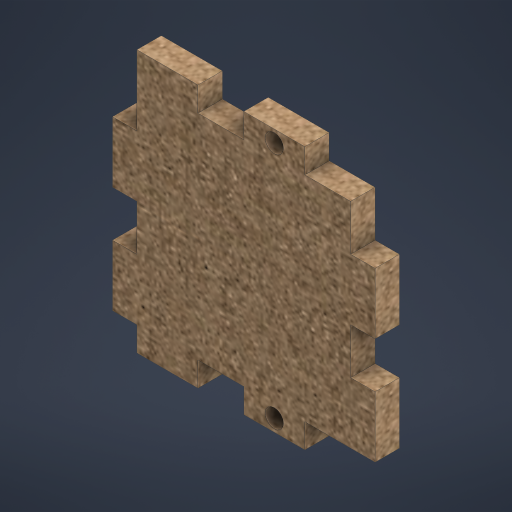
# Autodesk Inventor part: FloorButtonHolder_Back_V1
Saved by Autodesk Inventor 2024.1 (Build 281209000, 209)
## iProperties
Created: 2023-05-20
Part Number: FloorButtonHolder_Back_V1
Material: MDF Medium Density Fiberboard
Document SubType Name: Modeling
Designer: jaege
Density: 0.8 g/cm^3
Appearance: Cardboard - Corrugated
Author: jaege
Autodesk Inventor part; units mm, degrees
ref_plane "YZ Plane" through (0, 0, 0) normal (1, 0, 0) x (0, 1, 0)
ref_plane "XZ Plane" through (0, 0, 0) normal (0, 1, 0) x (-1, 0, 0)
ref_plane "XY Plane" through (0, 0, 0) normal (0, 0, 1) x (1, 0, 0)
sketch "Sketch1" plane through (0, 0, 0) normal (0, 0, 1) x (1, 0, 0)
  line L0 (17.5, -17.5) -> (0, -17.5)
  line L1 (-17.5, -17.5) -> (-17.5, 17.5)
  line L2 (-17.5, 17.5) -> (-7.5, 17.5) construction
  line L3 (17.5, 17.5) -> (17.5, 10)
  line L4 (17.5, -17.5) -> (-17.5, 17.5) construction
  line L5 (-17.5, -17.5) -> (17.5, 17.5) construction
  line L6 (-17.5, -17.5) -> (-21.5, -17.5)
  line L7 (-21.5, -17.5) -> (-21.5, -7.5)
  line L8 (-21.5, -7.5) -> (-17.5, -7.5)
  line L9 (-17.5, -7.5) -> (-17.5, -17.5) construction
  line L10 (-17.5, 0) -> (-21.5, 0)
  line L11 (-21.5, 0) -> (-21.5, 10)
  line L12 (-21.5, 10) -> (-17.5, 10)
  line L13 (-17.5, 10) -> (-17.5, 0) construction
  line L14 (-17.5, 17.5) -> (-7.5, 17.5) construction
  line L15 (-7.5, 17.5) -> (-7.5, 21.5)
  line L16 (-7.5, 21.5) -> (-17.5, 21.5)
  line L17 (-17.5, 21.5) -> (-17.5, 17.5)
  line L18 (0, 17.5) -> (10, 17.5) construction
  line L19 (10, 17.5) -> (10, 21.5)
  line L20 (10, 21.5) -> (0, 21.5)
  line L21 (0, 21.5) -> (0, 17.5)
  line L22 (-17.5, 0) -> (17.5, 0) construction
  line L23 (0, -17.5) -> (0, 17.5) construction
  line L24 (-17.5, -17.5) -> (-7.5, -17.5)
  line L25 (-7.5, -17.5) -> (-7.5, -21.5)
  line L26 (-7.5, -21.5) -> (-17.5, -21.5)
  line L27 (-17.5, -21.5) -> (-17.5, -17.5)
  line L28 (0, -17.5) -> (10, -17.5) construction
  line L29 (10, -17.5) -> (10, -21.5)
  line L30 (10, -21.5) -> (0, -21.5)
  line L31 (0, -21.5) -> (0, -17.5)
  line L32 (17.5, -17.5) -> (21.5, -17.5)
  line L33 (21.5, -17.5) -> (21.5, -7.5)
  line L34 (21.5, -7.5) -> (17.5, -7.5)
  line L35 (17.5, -7.5) -> (17.5, -17.5) construction
  line L36 (17.5, 0) -> (21.5, 0)
  line L37 (21.5, 0) -> (21.5, 10)
  line L38 (21.5, 10) -> (17.5, 10)
  line L39 (17.5, 10) -> (17.5, 0) construction
  line L40 (-7.5, 17.5) -> (0, 17.5)
  line L41 (0, 17.5) -> (10, 17.5)
  line L42 (17.5, 10) -> (17.5, 0) construction
  line L43 (17.5, 0) -> (17.5, -7.5)
  line L44 (17.5, -7.5) -> (17.5, -17.5) construction
  line L45 (0, -17.5) -> (-17.5, -17.5)
  line L46 (10, 17.5) -> (17.5, 17.5)
  point P0 (0, 0)
  point P1 (0, 19.5)
  point P2 (-7.5, 19.5)
  point P3 (0, -19.5)
  point P4 (-7.5, -19.5)
  point P5 (-17.5, -7.5)
  point P6 (10, -17.5)
  dimension "d5" = 10
  dimension "d6" = 10
  dimension "d7" = 7.5
  dimension "d8" = 4
  dimension "d9" = 10
  dimension "d10" = 4
  dimension "d11" = 10
  dimension "d12" = 4
  dimension "d13" = 7.5
  dimension "d16" = 35
  dimension "d17" = 35
  constraints: 94 end point, 20 parallel, 17 symmetric about line, 6 horizontal, 6 perpendicular, 5 midpoint, 3 collinear, 3 point on line
  measures "d5" distance of L10.end L11.end
  measures "d6" distance of L6.end L7.end
  measures "d7" distance between parallel lines of L8 L10
  measures "d8" distance of L11.end L12.end
  measures "d9" distance of L16.end L15.end
  measures "d10" distance of L15.end L2.end
  measures "d11" distance of L20.end L19.end
  measures "d12" distance of L19.end L18.end
  measures "d13" distance of point (0, 19.5) point (-7.5, 19.5)
  measures "d16" distance between parallel lines of L0 L40
  measures "d17" distance between parallel lines of L43 L1
extrude "Extrusion1" add sketch "Sketch1" along normal blind 4
sketch "Sketch2" plane through (0, 0, 0) normal (0, 0, -1) x (-1, 0, 0)
  line L0 (-3.5, 17.5) -> (-6.5, 17.5) construction
  line L1 (-3.5, 21.5) -> (-3.5, 17.5) construction
  line L2 (-6.5, 21.5) -> (-3.5, 21.5) construction
  line L3 (-6.5, 21.5) -> (-6.5, 17.5) construction
  line L4 (-3.5, -21.5) -> (-6.5, -21.5) construction
  line L5 (-3.5, -17.5) -> (-3.5, -21.5) construction
  line L6 (-6.5, -17.5) -> (-3.5, -17.5) construction
  line L7 (-6.5, -17.5) -> (-6.5, -21.5) construction
  line L8 (-6.5, 21.5) -> (-3.5, 17.5) construction
  line L9 (-6.5, -21.5) -> (-3.5, -17.5) construction
  circle A0 centre (-5, 19.5) radius 1.5
  circle A1 centre (-5, -19.5) radius 1.5
  point P0 (0, 0)
  dimension "d18" = 3
  constraints: 4 end point, 3 midpoint, 2 centre point, 1 equal radius
  measures "d18" diameter of A0
extrude "Extrusion2" cut sketch "Sketch2" against normal up to next
body "Solid1"
